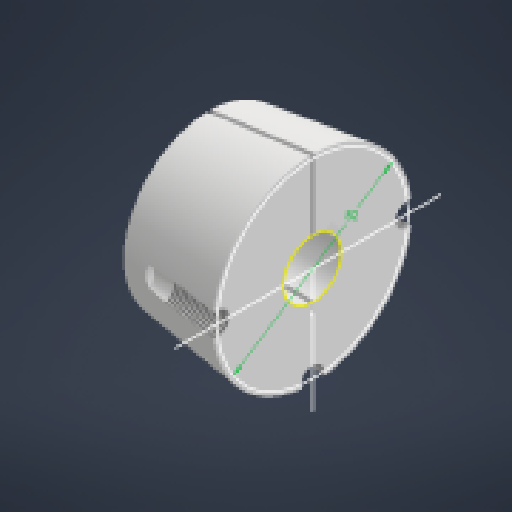
# Autodesk Inventor part: Douille2517
Saved by Autodesk Inventor 2026.2 (Build 302298010, 298A)
## iProperties
Created: 2026-04-10
Part Number: Douille2517
Material: Générique
Document SubType Name: Modeling
Designer: romai
Density: 1 g/cm^3
Appearance: Par défaut
Author: romai
Autodesk Inventor part; units mm, degrees
ref_plane "YZ Plane" through (0, 0, 0) normal (1, 0, 0) x (0, 1, 0)
ref_plane "XZ Plane" through (0, 0, 0) normal (0, 1, 0) x (-1, 0, 0)
ref_plane "XY Plane" through (0, 0, 0) normal (0, 0, 1) x (1, 0, 0)
sketch "Esquisse1" plane through (0, 0, 0) normal (0, 0, 1) x (1, 0, 0)
  line L0 (-36.1898, 0) -> (37.2521, 0)
  line L1 (0, 12.5) -> (-44.5, 12.5)
  line L2 (-44.5, 12.5) -> (-44.5, 36.75)
  line L3 (-44.5, 36.75) -> (0, 42.75)
  line L4 (0, 42.75) -> (0, 12.5)
  point P0 (0, 0)
  dimension "d0" = 25
  dimension "d1" = 85.5
  dimension "d2" = 0
  dimension "d3" = 73.5
  dimension "d4" = 44.5
  dimension "d5" = 0
  constraints: 10 end point, 2 horizontal, 1 parallel, 1 perpendicular
  measures "d0" diameter of L1 L0
  measures "d1" diameter of L3.end L0
  measures "d2" distance from line of point (0, 0) L0
  measures "d3" diameter of L2.end L0
  measures "d4" distance between parallel lines of L4 L2
  measures "d5" distance from line of point (0, 0) L4
revolve "Révolution1" add sketch "Esquisse1" angle 360 about axis through (-36.1898, 0, 0) along (1, 0, 0)
sketch "Esquisse3" plane through (0, 0, 0) normal (1, 0, 0) x (0, 0, -1)
  circle A0 centre (0, 0) radius 41
  circle A1 centre (0, 0) radius 12.5 projected
  line L0 (0, 0) -> (-59.2945, 0)
  line L1 (0, 0) -> (0, -53.2291)
  line L2 (0, 0) -> (55.0659, 0)
  point P0 (0, -41)
  point P1 (41, 0)
  point P2 (-41, 0)
  dimension "d16" = 82
  constraints: 6 end point, 3 point on circle, 3 point on line, 2 horizontal, 1 centre point, 1 coincident, 1 vertical
  measures "d16" diameter of A0
hole "Perçage1" at (0, -41, 0) at (0, 0, 41) at (0, 0, -41) direction (-1, 0, 0) diameter 10.106 depth 32.3 tip angle 118 thread size "M12x1.75" class "6H" standard "ANSI Metric M Profile"
sketch "Esquisse4" plane through (0, 0, 0) normal (1, 0, 0) x (0, 0, 1)
  line L0 (0, 0) -> (-39.036, -39.036)
  line L1 (0, 0) -> (-55.3193, 0)
  circle A0 centre (0, 0) radius 12.5 projected
  line L2 (-5.5456, -11.2025) -> (-7.8791, -13.5359)
  line L3 (-11.2025, -5.5456) -> (-13.5359, -7.8791)
  line L4 (-13.5359, -7.8791) -> (-7.8791, -13.5359)
  dimension "d17" = 45
  dimension "d20" = 3.3
  dimension "d21" = 3.3
  dimension "d22" = 4
  dimension "d23" = 4
  constraints: 10 end point, 2 parallel, 2 point on circle, 1 horizontal
  measures "d17" angle of L1 L0
  measures "d20" distance of L2.start L2.end
  measures "d21" distance of L3.start L3.end
  measures "d22" distance between parallel lines of L0 L3
  measures "d23" distance between parallel lines of L0 L2
extrude "Extrusion1" cut sketch "Esquisse4" against normal through all contours A0 L2 L4 L0 | L0 L4 L3 A0
sketch "Esquisse5" plane through (0, 0, 0) normal (1, 0, 0) x (0, 0, 1)
  line L0 (-1, 17.25) -> (1, 17.25)
  line L1 (1, 17.25) -> (1, -42.75)
  line L2 (1, -42.75) -> (-1, -42.75)
  line L3 (-1, -42.75) -> (-1, 17.25)
  line L4 (-1, 17.25) -> (1, -42.75) construction
  line L5 (1, 17.25) -> (-1, -42.75) construction
  arc A0 (-4.8326, 42.476) -> (4.8326, 42.476) centre (0, 0) ccw projected
  point P0 (0, -12.75)
  point P1 (42.6948, 2.1722)
  point P2 (-42.6948, 2.1722)
  point P3 (4.9266, -42.4652)
  point P4 (42.5102, -4.5219)
  dimension "d26" = 2
  dimension "d27" = 60
  dimension "d28" = 0
  constraints: 12 end point, 2 midpoint, 2 parallel, 1 horizontal, 1 perpendicular, 1 tangent
  measures "d26" distance of L1.end L2.end
  measures "d27" distance of L0.end L1.end
  measures "d28" horizontal distance of point (0, 0) point (0, -12.75)
extrude "Extrusion2" cut sketch "Esquisse5" against normal through all
